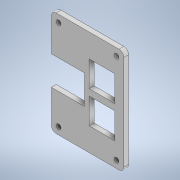
# Autodesk Inventor part: level2_up
Saved by Autodesk Inventor 2021.2 (Build 252289000, 289)
## iProperties
Created: 2021-11-19
Part Number: level2_up
Material: Типовые
Document SubType Name: Modeling
Designer: kanad
Density: 1 g/cm^3
Appearance: По умолчанию
Author: kanad
Autodesk Inventor part; units mm, degrees
ref_plane "YZ Plane" through (0, 0, 0) normal (1, 0, 0) x (0, 1, 0)
ref_plane "XZ Plane" through (0, 0, 0) normal (0, 1, 0) x (-1, 0, 0)
ref_plane "XY Plane" through (0, 0, 0) normal (0, 0, 1) x (1, 0, 0)
sketch "Эскиз1" plane through (0, 0, 0) normal (0, 0, 1) x (1, 0, 0)
  arc A0 (22.5, 29.5) -> (19.5, 32.5) centre (19.5, 29.5) ccw projected
  line L0 (22.5, -29.5) -> (22.5, 29.5) projected
  arc A1 (19.5, -32.5) -> (22.5, -29.5) centre (19.5, -29.5) ccw projected
  line L1 (-19.5, -32.5) -> (19.5, -32.5) projected
  line L2 (19.5, 32.5) -> (-19.5, 32.5) projected
  arc A2 (-19.5, 32.5) -> (-22.5, 29.5) centre (-19.5, 29.5) ccw projected
  line L3 (-22.5, 29.5) -> (-22.5, 9) projected
  line L4 (-22.5, -9) -> (-22.5, -29.5) projected
  arc A3 (-22.5, -29.5) -> (-19.5, -32.5) centre (-19.5, -29.5) ccw projected
  circle A4 centre (-18, -28) radius 1.5 projected
  circle A5 centre (18, -28) radius 1.5 projected
  circle A6 centre (18, 28) radius 1.5 projected
  circle A7 centre (-18, 28) radius 1.5 projected
  line L5 (-2, 9) -> (-20, 9) projected
  line L6 (-22.5, 9) -> (-20, 9) projected
  line L7 (-2, -9) -> (-2, 9) projected
  line L8 (-20, -9) -> (-2, -9) projected
  line L9 (-20, -9) -> (-22.5, -9) projected
  line L10 (1, -2) -> (1, -18) projected
  line L11 (1, -18) -> (17, -18) projected
  line L12 (17, -18) -> (17, -2) projected
  line L13 (17, -2) -> (1, -2) projected
  line L14 (1, 18) -> (1, 2) projected
  line L15 (1, 2) -> (17, 2) projected
  line L16 (17, 2) -> (17, 18) projected
  line L17 (17, 18) -> (1, 18) projected
  point P0 (0, 0)
extrude "Выдавливание1" add sketch "Эскиз1" along normal blind 3
